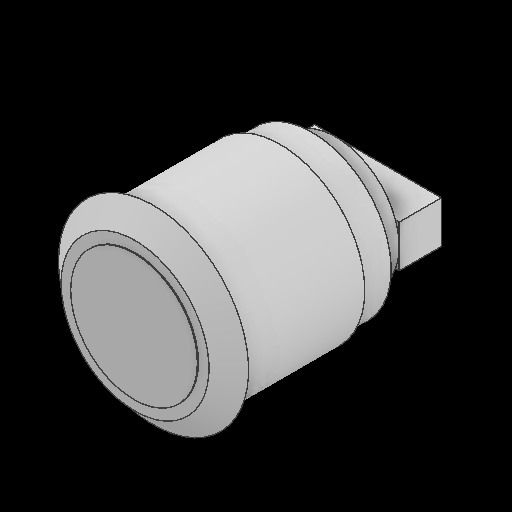
# Autodesk Inventor part: PilotLight
Saved by Autodesk Inventor 2025.2 (Build 292293000, 293)
## iProperties
Created: 2026-05-14
Part Number: PilotLight
Material: Generic
Document SubType Name: Modeling
Designer: valer
Density: 1 g/cm^3
Appearance: Default
Author: valer
Autodesk Inventor part; units mm, degrees
ref_plane "YZ Plane" through (0, 0, 0) normal (1, 0, 0) x (0, 1, 0)
ref_plane "XZ Plane" through (0, 0, 0) normal (0, 1, 0) x (-1, 0, 0)
sketch "BaseBottom" plane through (0, 0, 0) normal (0, 0, 1) x (1, 0, 0)
  circle A0 centre (0, 0) radius 9
  dimension "d0" = 18
  constraints: 1 centre point, 1 coincident
  measures "d0" diameter of A0
ref_plane "TopPlane" through (0, 0, 1.75) normal (0, 0, 1) x (1, 0, 0)
sketch "BaseTop" plane through (0, 0, 1.75) normal (0, 0, 1) x (1, 0, 0)
  circle A0 centre (0, 0) radius 7
  dimension "d4" = 14
  constraints: 1 centre point, 1 coincident
  measures "d4" diameter of A0
loft "BaseFeature" add profiles "BaseBottom", "BaseTop"
sketch "Light" plane through (0, 0, 1.75) normal (0, 0, 1) x (1, 0, 0)
  circle A0 centre (0, 0) radius 9 projected
  circle A1 centre (0, 0) radius 6
  dimension "d9" = 12
  constraints: 1 centre point, 1 coincident
  measures "d9" diameter of A1
extrude "LightFeature" add sketch "Light" along normal blind 0.1 contours A1
sketch "Thread" plane through (0, 0, 0) normal (0, 0, -1) x (-1, 0, 0)
  circle A0 centre (0, 0) radius 8
  dimension "d12" = 16
  constraints: 1 centre point, 1 coincident
  measures "d12" diameter of A0
extrude "ThreadFeature" add sketch "Thread" along normal blind 12
sketch "Body" plane through (0, 0, -12) normal (0, 0, -1) x (-1, 0, 0)
  circle A0 centre (0, 0) radius 7.5
  dimension "d15" = 15
  constraints: 1 centre point, 1 coincident
  measures "d15" diameter of A0
extrude "BodyFeature" add sketch "Body" along normal blind 3
sketch "TerminalsBase" plane through (0, 0, -15) normal (0, 0, -1) x (-1, 0, 0)
  circle A0 centre (0, 0) radius 6
  dimension "d18" = 12
  constraints: 1 centre point, 1 coincident
  measures "d18" diameter of A0
extrude "TerminalsBaseFeature" add sketch "TerminalsBase" along normal blind 2.25
sketch "Terminals" plane through (0, 0, -17.25) normal (0, 0, -1) x (-1, 0, 0)
  line L0 (-6, -2) -> (6, -2)
  line L1 (6, -2) -> (6, 2)
  line L2 (6, 2) -> (-6, 2)
  line L3 (-6, 2) -> (-6, -2)
  line L4 (-6, -2) -> (6, 2) construction
  line L5 (6, -2) -> (-6, 2) construction
  circle A0 centre (0, 0) radius 6 projected
  dimension "d21" = 4
  constraints: 12 end point, 2 midpoint, 2 parallel, 1 horizontal, 1 perpendicular, 1 tangent
  measures "d21" distance of L2.end L0.start
extrude "TerminalsFeature" add sketch "Terminals" along normal blind 4 contours L3 A0 L0 | A0 L2 L0 | L3 L2 A0 | A0 L1 L0 | A0 L2 L1
body "Solid2"
